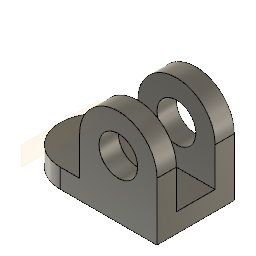
tut 1_ P4 (Autodesk Fusion 360 design; units mm, degrees)
Autodesk Fusion 360 part; units mm, degrees
sketch "Sketch1" plane through (0, 0, 0) normal (0, 1, 0) x (1, 0, 0)
  line L0 (0, 0) -> (0, -12.7)
  line L1 (0, -12.7) -> (38.1, -12.7)
  line L2 (38.1, -12.7) -> (38.1, -38.1)
  line L3 (0, 0) -> (88.9, 0)
  line L4 (88.9, 0) -> (88.9, -38.1)
  arc A0 (38.1, -38.1) -> (88.9, -38.1) centre (63.5, -38.1) ccw
  circle A1 centre (63.5, -38.1) radius 12.7
extrude "Extrude1" add sketch "Sketch1" along normal mid plane 50.8
sketch "Sketch2" plane through (88.9, 0, 0) normal (1, 0, 0) x (0, 1, 0)
  line L0 (-25.4, 0) -> (25.4, 0)
  line L1 (25.4, 0) -> (25.4, 38.1)
  line L2 (25.4, 38.1) -> (-25.4, 38.1)
  line L3 (-25.4, 38.1) -> (-25.4, 0)
  line L4 (-12.7, 67.4271) -> (-12.7, 12.7)
  line L5 (-12.7, 12.7) -> (12.7, 12.7)
  line L6 (12.7, 12.7) -> (12.7, 67.4271)
  line L7 (-12.7, 63.5) -> (12.7, 63.5)
  dimension "d3" = 12.7
  dimension "d4" = 12.7
  dimension "d5" = 12.7
  measures "d3" distance of L3 L4
  measures "d4" distance of L1 L6
  measures "d5" distance of L0 L5
extrude "Extrude2" cut sketch "Sketch2" against normal blind 50.8 contours L2 L4 L6 L7 | L2 L4 L5 L6
sketch "Sketch3" plane through (0, 0, 0) normal (-1, 0, 0) x (0, -1, 0)
  line L0 (25.4, 12.7) -> (-25.4, 12.7)
  line L1 (-25.4, 12.7) -> (-25.4, 0)
  line L2 (-25.4, 0) -> (25.4, 0)
  line L3 (25.4, 0) -> (25.4, 12.7)
fillet "Fillet1" radius 25.4 1 edges at (0, -25.4, 6.35)
fillet "Fillet2" radius 25.4 1 edges at (0, 25.4, 6.35)
